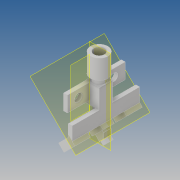
# Autodesk Inventor part: LickSensorMount
Saved by Autodesk Inventor 2020 (Build 240168000, 168)
## iProperties
Created: 2019-07-29
Part Number: LickSensorMount
Material: 일반
Document SubType Name: Modeling
Designer: Jeong Ji Hoon
Density: 1 g/cm^3
Appearance: 기본값
Author: Jeong Ji Hoon
## iProperties of the stored document LickSensorMount_3D 인쇄.ipt
Created: 2019-07-29
Part Number: LickSensorMount_3D 인쇄
Material: 일반
Document SubType Name: Modeling
Designer: Jeong Ji Hoon
Density: 1 g/cm^3
Appearance: 기본값
Author: Jeong Ji Hoon
Autodesk Inventor part; units mm, degrees
ref_plane "YZ Plane" through (0, 0, 0) normal (1, 0, 0) x (0, 1, 0)
ref_plane "XZ Plane" through (0, 0, 0) normal (0, 1, 0) x (-1, 0, 0)
ref_plane "XY Plane" through (0, 0, 0) normal (0, 0, 1) x (1, 0, 0)
sketch "스케치1" plane through (0, 0, 0) normal (0, 1, 0) x (-1, 0, 0)
  line L0 (0, 0) -> (7, 0)
  line L1 (7, 0) -> (7, -7)
  line L2 (7, -7) -> (0, -7)
  line L3 (0, -7) -> (0, 0)
  dimension "d0" = 7
  dimension "d1" = 7
  constraints: 8 end point, 2 parallel, 1 horizontal, 1 perpendicular
  measures "d0" distance of L1.end L2.end
  measures "d1" distance of L0.end L1.end
extrude "돌출1" add sketch "스케치1" along normal blind 10
sketch "스케치2" plane through (0, 10, 0) normal (0, 1, 0) x (1, 0, 0)
  line L0 (-7, 0) -> (0, 0) projected
  line L1 (0, 0) -> (0, 7) projected
  line L2 (0, 7) -> (-7, 7) projected
  line L3 (-7, 7) -> (-7, 0) projected
  circle A0 centre (-3.5, 3.5) radius 3
  line L4 (-7, 3.5) -> (0, 3.5) construction
  line L5 (-3.5, 7) -> (-3.5, 0) construction
  point P0 (-3.5, 3.5)
  dimension "d4" = 6
  constraints: 5 midpoint, 4 end point, 1 centre point, 1 coincident
  measures "d4" diameter of A0
extrude "돌출2" add sketch "스케치2" along normal blind 3 contours A0
sketch "스케치3" plane through (-3.5, 13, -3.5) normal (0, 1, 0) x (1, 0, 0)
  circle A0 centre (0, 0) radius 3 projected
  circle A1 centre (0, 0) radius 4.5
  point P0 (3.5, -3.5)
  dimension "d7" = 9
  constraints: 1 centre point, 1 coincident
  measures "d7" diameter of A1
extrude "돌출3" add sketch "스케치3" along normal blind 10 contours A0 | A1
ref_plane "작업 평면1" through (-3.5, 0, 0) normal (1, 0, 0) x (0, 0, -1)
sketch "스케치4" plane through (-3.5, 0, 0) normal (1, 0, 0) x (0, 0, -1)
  line L0 (8, 23) -> (-1, 23) projected
  line L1 (-1, 13) -> (8, 13) projected
  line L2 (3.5, 23) -> (3.5, 13) construction
  line L3 (3.5, 23) -> (0.75, 23)
  line L4 (0.75, 23) -> (0.75, 18)
  line L5 (0.75, 18) -> (3, 15.5)
  line L6 (3, 15.5) -> (3, 13)
  line L7 (3, 13) -> (3.5, 13)
  line L8 (3.5, 13) -> (3.5, 23)
  point P0 (0, 0)
  dimension "d10" = 2.75
  dimension "d11" = 5
  dimension "d12" = 2.5
  dimension "d13" = 0.5
  constraints: 14 end point, 2 collinear, 2 midpoint, 2 point on line, 1 parallel, 1 vertical
  measures "d10" distance of L2.start L3.end
  measures "d11" distance of L3.end L4.end
  measures "d12" vertical distance of L5.end L4.end
  measures "d13" distance between parallel lines of L6 L2
revolve "회전2" cut sketch "스케치4" angle 360 about axis through (-3.5, 13, -3.5) along (0, 1, 0)
sketch "스케치5" plane through (0, 0, 0) normal (1, 0, 0) x (0, 0, -1)
  line L0 (7, 0) -> (0, 0) projected
  line L1 (-14, -7) -> (21, -7)
  line L2 (21, -7) -> (21, 0)
  line L3 (21, 0) -> (-14, 0)
  line L4 (-14, 0) -> (-14, -7)
  point P0 (3.5, 0)
  dimension "d16" = 35
  dimension "d17" = 7
  constraints: 8 end point, 2 midpoint, 2 parallel, 1 horizontal, 1 perpendicular
  measures "d16" distance of L1.start L1.end
  measures "d17" distance of L3.end L1.start
extrude "돌출4" add sketch "스케치5" against normal blind 2
sketch "스케치6" plane through (0, 0, 0) normal (0, -1, 0) x (1, 0, 0)
  circle A0 centre (-3.5, -3.5) radius 2.5
  circle A1 centre (-3.5, -3.5) radius 0.5 projected
  point P0 (0, 0)
  dimension "d20" = 5
  constraints: 2 coincident, 1 centre point
  measures "d20" diameter of A0
extrude "돌출5" add sketch "스케치6" along normal blind 11 contours A0 | A1
ref_plane "작업 평면2" through (0, -7, 0) normal (0.7071068, 0.7071068, 0) x (0, 0, 1)
sketch "스케치7" plane through (0, -7, 0) normal (0.7071068, 0.7071068, 0) x (0, 0, 1)
  line L0 (-7, -4.9497) -> (-7, -12.0208) projected
  line L1 (0, -12.0208) -> (-7, -12.0208) projected
  line L2 (0, -4.9497) -> (0, -12.0208) projected
  line L3 (0, -4.9497) -> (14, -4.9497) projected
  line L4 (14, -4.9497) -> (14, 0) projected
  line L5 (14, 0) -> (-21, 0) projected
  line L6 (-21, 0) -> (-21, -4.9497) projected
  line L7 (-21, -4.9497) -> (-7, -4.9497) projected
  line L8 (-21, 2) -> (14, 2)
  line L9 (14, 2) -> (14, -2)
  line L10 (14, -2) -> (-21, -2)
  line L11 (-21, -2) -> (-21, 2)
  dimension "d23" = 35
  dimension "d24" = 4
  dimension "d25" = 2
  constraints: 8 end point, 2 parallel, 1 collinear, 1 horizontal, 1 perpendicular
  measures "d23" distance of L9.end L10.end
  measures "d24" distance of L8.end L9.end
  measures "d25" distance between parallel lines of L8 L5
extrude "돌출6" add sketch "스케치7" against normal blind 8 contours L6 L5 L4 L10 | L11 L8 L9 L5
sketch "스케치8" plane through (1.4142, -8.4142, 14) normal (0.7071068, -0.7071068, 0) x (-0.7071068, -0.7071068, 0)
  line L0 (0, 35) -> (0, 0) projected
  line L1 (0, 0) -> (8, 0) projected
  line L2 (8, 35) -> (8, 0) projected
  line L3 (0, 35) -> (8, 35) projected
  line L4 (1, 1.5) -> (7, 1.5)
  line L5 (7, 1.5) -> (7, 6.1)
  line L6 (7, 6.1) -> (1, 6.1)
  line L7 (1, 6.1) -> (1, 1.5)
  line L8 (1, 28.9) -> (7, 28.9)
  line L9 (7, 28.9) -> (7, 33.5)
  line L10 (7, 33.5) -> (1, 33.5)
  line L11 (1, 33.5) -> (1, 28.9)
  line L12 (8, 8.1) -> (0, 8.1)
  line L13 (8, 26.9) -> (0, 26.9)
  line L14 (8, 14.6) -> (0, 14.6)
  line L15 (8, 20.4) -> (0, 20.4)
  point P0 (-4.9497, 14)
  dimension "d28" = 6
  dimension "d29" = 4.6
  dimension "d30" = 4.6
  dimension "d31" = 1.5
  dimension "d32" = 1
  dimension "d33" = 1.5
  dimension "d34" = 2
  dimension "d35" = 2
  dimension "d36" = 6.5
  dimension "d37" = 6.5
  constraints: 24 end point, 10 point on line, 5 parallel, 5 perpendicular, 2 horizontal
  measures "d28" distance of L5.end L6.end
  measures "d29" distance of L4.end L5.end
  measures "d30" distance of L8.end L9.end
  measures "d31" distance between parallel lines of L1 L4
  measures "d32" distance between parallel lines of L2 L5
  measures "d33" distance between parallel lines of L3 L10
  measures "d34" distance between parallel lines of L6 L12
  measures "d35" distance between parallel lines of L8 L13
  measures "d36" distance between parallel lines of L12 L14
  measures "d37" distance between parallel lines of L13 L15
extrude "돌출7" cut sketch "스케치8" against normal through all contours L13 L2 L15 L0 | L14 L2 L12 L0 | L7 L6 L5 L4 | L11 L10 L9 L8
sketch "스케치9" plane through (1.4142, -8.4142, -0.6) normal (0.7071068, -0.7071068, 0) x (-0.7071068, -0.7071068, 0)
  ellipse E0 centre (6.9497, 2.9) end of major axis (10.4853, 2.9) minor radius 2.5 (3.6569, 3.8102) -> (3.6569, 1.9898) ccw projected
  line L0 (3.6569, 1.9898) -> (3.6569, 3.8102) projected
  line L1 (8, 5.8) -> (8, 0) projected
  line L2 (0, 5.8) -> (0, 0) projected
  line L3 (2, 0.9) -> (7, 0.9)
  line L4 (7, 0.9) -> (7, 4.9)
  line L5 (7, 4.9) -> (2, 4.9)
  line L6 (2, 4.9) -> (2, 0.9)
  line L7 (8, 2.9) -> (0, 2.9) construction
  point P0 (-4.9497, -0.6)
  point P1 (2, 2.9)
  dimension "d40" = 4
  dimension "d41" = 5
  dimension "d42" = 1
  constraints: 10 end point, 3 midpoint, 2 parallel, 1 horizontal, 1 perpendicular, 1 point on line, 1 other
  measures "d40" distance of L3.end L4.end
  measures "d41" distance of L4.end L5.end
  measures "d42" distance between parallel lines of L4 L1
extrude "돌출8" add sketch "스케치9" along normal blind 3 contours L0 E0 | L6 L5 L4 L3
sketch "스케치10" plane through (3.5355, -10.5355, -0.6) normal (0.7071068, -0.7071068, 0) x (0, 0, -1)
  line L0 (0.9, -2) -> (0.9, -7) projected
  line L1 (0.9, -7) -> (4.9, -7) projected
  line L2 (4.9, -7) -> (4.9, -2) projected
  line L3 (1.15, -4) -> (4.65, -4)
  line L4 (4.65, -4) -> (4.65, -6.5)
  line L5 (4.65, -6.5) -> (1.15, -6.5)
  line L6 (1.15, -6.5) -> (1.15, -4)
  point P0 (-0.6, 4.9497)
  dimension "d45" = 3.5
  dimension "d46" = 2.5
  dimension "d47" = 0.5
  dimension "d48" = 0.25
  dimension "d49" = 0.25
  constraints: 8 end point, 2 parallel, 1 horizontal, 1 perpendicular
  measures "d45" distance of L4.end L5.end
  measures "d46" distance of L3.end L4.end
  measures "d47" distance between parallel lines of L5 L1
  measures "d48" distance between parallel lines of L0 L6
  measures "d49" distance between parallel lines of L2 L4
extrude "돌출9" add sketch "스케치10" along normal blind 2
sketch "스케치11" plane through (4.9497, -11.9497, -0.6) normal (0.7071068, -0.7071068, 0) x (-0.7071068, -0.7071068, 0)
  line L0 (4, 4.65) -> (4, 1.15) projected
  line L1 (4, 1.15) -> (6.5, 1.15) projected
  line L2 (6.5, 1.15) -> (6.5, 4.65) projected
  line L3 (6.5, 4.65) -> (4, 4.65) projected
  line L4 (4.5, 1.65) -> (4.5, 4.15)
  line L5 (4.5, 4.15) -> (6, 4.15)
  line L6 (6, 4.15) -> (6, 1.65)
  line L7 (6, 1.65) -> (4.5, 1.65)
  point P0 (-4.9497, -0.6)
  dimension "d52" = 0.5
  constraints: 8 end point, 3 other
  measures "d52" distance between parallel lines of L0 L4
extrude "돌출10" cut sketch "스케치11" against normal blind 8 contours L4 L5 L6 L7
ref_plane "작업 평면3" through (-7, 10, -3.5) normal (0, 0, 1) x (1, 0, 0)
chamfer "모따기1" distance 2 angle 45 1 edges at (2.1213, -11.9497, -3.5)
sketch "스케치13" plane through (-2, -6.1716, 5.9) normal (0, 0, -1) x (-1, 0, 0)
  line L0 (0, 1.1716) -> (0, 0) projected
  line L1 (0, 0) -> (5.0711, -5.0711) projected
  line L2 (5.0711, -5.0711) -> (2.2426, -7.8995) projected
  line L3 (2.2426, -7.8995) -> (-3.4142, -2.2426) projected
  line L4 (-3.4142, -2.2426) -> (-2, -0.8284) projected
  line L5 (0, 1.1716) -> (-2, -0.8284) projected
  line L6 (0, 6.1716) -> (0, 1.1716) projected
  line L7 (-2, 6.1716) -> (0, 6.1716) projected
  line L8 (-2, -0.8284) -> (-2, 6.1716) projected
  line L9 (0, 0) -> (5.0711, -5.0711) projected
  line L10 (0, 1.1716) -> (0, 0) projected
  line L11 (0, 6.1716) -> (5.0711, -5.0711)
  constraints: 2 end point
extrude "돌출12" add sketch "스케치13" against normal up to surface (2 mm away) contours L6 L11 L1 L0
sketch "스케치14" plane through (-2, -6.1716, -12.9) normal (0, 0, 1) x (1, 0, 0)
  line L0 (-2.2426, -7.8995) -> (-5.0711, -5.0711) projected
  line L1 (-5.0711, -5.0711) -> (0, 0) projected
  line L2 (0, 0) -> (0, 1.1716) projected
  line L3 (2, -0.8284) -> (0, 1.1716) projected
  line L4 (2, -0.8284) -> (3.4142, -2.2426) projected
  line L5 (3.4142, -2.2426) -> (-2.2426, -7.8995) projected
  line L6 (0, 1.1716) -> (0, 6.1716) projected
  line L7 (0, 6.1716) -> (2, 6.1716) projected
  line L8 (2, 6.1716) -> (2, -0.8284) projected
  line L9 (0, 6.1716) -> (-5.0711, -5.0711)
  constraints: 2 end point
extrude "돌출13" add sketch "스케치14" against normal up to surface (2 mm away) contours L9 L6 L2 L1
sketch "스케치15" plane through (-3.5, 23, -3.5) normal (0, 1, 0) x (1, 0, 0)
  circle A0 centre (0, 0) radius 4.5 projected
  circle A1 centre (0, 0) radius 0.5
  point P0 (3.5, -3.5)
  dimension "d68" = 1
  constraints: 1 centre point, 1 coincident
  measures "d68" diameter of A1
extrude "돌출14" cut sketch "스케치15" against normal up to next contours A1
sketch "스케치16" plane through (-7, 0, 0) normal (-1, 0, 0) x (0, 0, 1)
  line L0 (0, 0) -> (-7, 0) projected
  line L1 (0, 0) -> (0, 10) projected
  line L2 (-7, 10) -> (0, 10) projected
  line L3 (-7, 0) -> (-7, 10) projected
  line L4 (11.5, 10) -> (-18.5, 10)
  line L5 (-18.5, 10) -> (-18.5, 2)
  line L6 (-18.5, 2) -> (11.5, 2)
  line L7 (11.5, 2) -> (11.5, 10)
  point P0 (-3.5, 10)
  dimension "d71" = 30
  dimension "d82" = 8
  constraints: 8 end point, 2 midpoint, 2 parallel, 1 collinear, 1 horizontal, 1 perpendicular
  measures "d71" distance of L5.end L6.end
  measures "d82" distance of L6.end L4.start
extrude "돌출15" add sketch "스케치16" against normal blind 2 contours L1 L4 L7 L6 | L6 L5 L4 L3
sketch "스케치17" plane through (-5, 0, 0) normal (1, 0, 0) x (0, 0, -1)
  line L0 (18.5, 2) -> (18.5, 10) projected
  line L1 (0, 0) -> (7, 0) projected
  line L2 (-11.5, 2) -> (-11.5, 10) projected
  line L3 (-11.5, 10) -> (18.5, 10) projected
  line L4 (18.5, 10) -> (18.5, 2) projected
  circle A0 centre (-5.75, 6) radius 2
  circle A1 centre (12.75, 6) radius 2
  line L5 (0, 0) -> (0, 2) projected
  line L6 (0, 2) -> (-11.5, 2) projected
  line L7 (18.5, 2) -> (7, 2) projected
  line L8 (7, 0) -> (7, 2) projected
  dimension "d74" = 4
  dimension "d75" = 4
  dimension "d76" = 5.75
  dimension "d77" = 5.75
  dimension "d81" = 4
  constraints: 2 centre point, 1 horizontal alignment
  measures "d74" diameter of A0
  measures "d75" diameter of A1
  measures "d76" distance from line of L0 A1.centre
  measures "d77" distance from line of L2 A0.centre
  measures "d81" distance from line of L3 A0.centre
extrude "돌출16" cut sketch "스케치17" against normal through all contours A0 | A1
